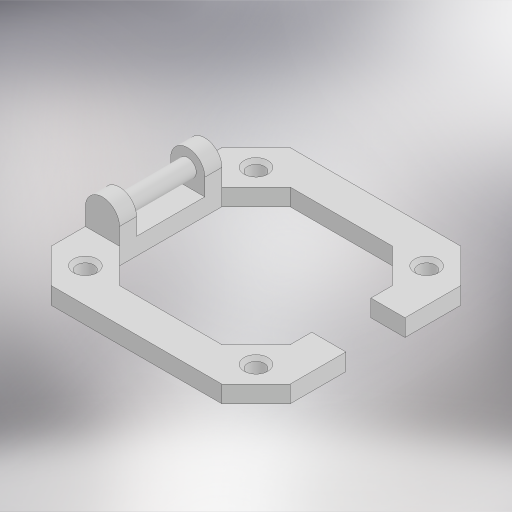
# Autodesk Inventor part: pokemon_ball_black_part1
Saved by Autodesk Inventor 2024 (Build 280153000, 153)
## iProperties
Created: 2023-10-25
Part Number: pokemon_ball_black_part1
Material: Generic
Document SubType Name: Modeling
Designer: SSAFY
Density: 1 g/cm^3
Appearance: Default
Author: SSAFY
Autodesk Inventor part; units mm, degrees
ref_plane "YZ Plane" through (0, 0, 0) normal (1, 0, 0) x (0, 1, 0)
ref_plane "XZ Plane" through (0, 0, 0) normal (0, 1, 0) x (-1, 0, 0)
ref_plane "XY Plane" through (0, 0, 0) normal (0, 0, 1) x (1, 0, 0)
sketch "Sketch2" plane through (0, 0, 0) normal (0, 1, 0) x (-1, 0, 0)
  line L0 (35, -35) -> (-35, -35)
  line L1 (-35, -35) -> (-35, 35)
  line L2 (-35, 35) -> (35, 35)
  line L3 (35, 35) -> (35, -35)
  line L4 (35, -35) -> (-35, 35) construction
  line L5 (-35, -35) -> (35, 35) construction
  line L6 (25, 25) -> (-25, 25)
  line L7 (-25, 25) -> (-25, -25)
  line L8 (-25, -25) -> (25, -25)
  line L9 (25, -25) -> (25, 25)
  point P0 (0, 0)
  dimension "d0" = 70
  dimension "d1" = 10
  dimension "d27" = 70
  constraints: 20 end point, 4 parallel, 2 midpoint, 2 perpendicular, 1 horizontal, 3 other
  measures "d0" distance of L1.end L2.end
  measures "d1" distance between parallel lines of L6 L2
  measures "d27" distance of L2.end L0.start
extrude "Extrusion1" add sketch "Sketch2" along normal blind 5
chamfer "Chamfer1" distance 10 angle 45 8 edges at (-25, 2.5, 25) (25, 2.5, 25) (-25, 2.5, -25) (25, 2.5, -25) (-35, 2.5, 35) (35, 2.5, 35) (35, 2.5, -35) (-35, 2.5, -35)
sketch "Sketch3" plane through (0, 5, 0) normal (0, 1, 0) x (1, 0, 0)
  line L0 (-35, 25) -> (-35, -25) construction
  line L1 (25, 35) -> (-25, 35) construction
  circle A0 centre (-25, 25) radius 2.5
  point P0 (0, 0)
  dimension "d7" = 10
  dimension "d8" = 10
  dimension "d9" = 5
  constraints: 1 centre point
  measures "d7" distance from line of A0.centre L0
  measures "d8" distance from line of L1 A0.centre
  measures "d9" diameter of A0
extrude "Extrusion2" cut sketch "Sketch3" against normal through all
pattern_circular "Circular Pattern1" count 4 over 360 about axis through (0, -10, 0) along (0, 1, 0) of "Extrusion2"
sketch "Sketch4" plane through (0, 0, 0) normal (0, 0, 1) x (1, 0, 0)
  line L0 (-35, 5) -> (-35, 0) construction
  line L1 (-35, 5) -> (-25, 5)
  line L2 (-25, 5) -> (-25, 15)
  line L3 (-25, 15) -> (-35, 15)
  line L4 (-35, 15) -> (-35, 5)
  point P0 (0, 0)
  dimension "d15" = 10
  dimension "d16" = 10
  constraints: 8 end point, 2 parallel, 1 horizontal, 1 perpendicular
  measures "d15" distance of L2.end L3.end
  measures "d16" distance of L1.end L2.end
extrude "Extrusion3" add sketch "Sketch4" along normal mid plane 30
sketch "Sketch6" plane through (0, 0, 0) normal (0, 0, 1) x (1, 0, 0)
  circle A0 centre (-30, 10) radius 2.5
  line L0 (-25, 15) -> (-35, 15) construction
  line L1 (-35, 15) -> (-35, 5) construction
  line L2 (-27.5, 5) -> (-22.5, 5) construction
  line L3 (-35, 15) -> (-25, 15)
  line L4 (-25, 15) -> (-25, 5)
  line L5 (-25, 5) -> (-35, 5)
  line L6 (-35, 5) -> (-35, 15)
  point P0 (0, 0)
  point P1 (-30, 15)
  point P2 (-35, 10)
  dimension "d22" = 5
  dimension "d23" = 5
  dimension "d24" = 5
  constraints: 8 end point, 3 midpoint, 2 parallel, 1 centre point, 1 horizontal, 1 perpendicular
  measures "d22" distance of point (-30, 15) A0.centre
  measures "d23" distance of point (-35, 10) A0.centre
  measures "d24" diameter of A0
extrude "Extrusion4" cut sketch "Sketch6" along normal mid plane 20
sketch "Sketch7" plane through (35, 0, 25) normal (1, 0, 0) x (0, 0, -1)
  line L0 (50, 5) -> (50, 0) construction
  line L1 (16.3397, 5) -> (25, 10)
  line L2 (25, 10) -> (33.6603, 5)
  line L3 (33.6603, 5) -> (33.6603, -5)
  line L4 (33.6603, -5) -> (25, -10)
  line L5 (25, -10) -> (16.3397, -5)
  line L6 (16.3397, -5) -> (16.3397, 5)
  point P0 (25, 0)
  point P1 (25, 0)
  dimension "d28" = 10
  constraints: 12 end point, 1 coincident, 1 parallel, 13 other
  measures "d28" distance of L2.end L3.end
extrude "Extrusion5" cut sketch "Sketch7" against normal blind 10
fillet "Fillet1" radius 5 4 edges at (-35, 15, 12.5) (-25, 15, 12.5) (-35, 15, -12.5) (-25, 15, -12.5)
chamfer "Chamfer2" distance 1 angle 45 4 edges at (-25, 5, 27.5) (-27.5, 5, -25) (25, 5, -27.5) (27.5, 5, 25)
body "Solid1"
